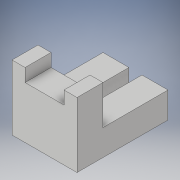
# Autodesk Inventor part: AddSub (1)
Saved by Autodesk Inventor 2019 (Build 230136000, 136)
## iProperties
Created: 2019-09-05
Part Number: AddSub (1)
Material: Generic
Document SubType Name: Modeling
Designer: IED8
Density: 1 g/cm^3
Appearance: Default
Author: IED8
Autodesk Inventor part; units mm, degrees
ref_plane "YZ Plane" through (0, 0, 0) normal (1, 0, 0) x (0, 1, 0)
ref_plane "XZ Plane" through (0, 0, 0) normal (0, 1, 0) x (-1, 0, 0)
ref_plane "XY Plane" through (0, 0, 0) normal (0, 0, 1) x (1, 0, 0)
sketch "Sketch1" plane through (0, 0, 0) normal (1, 0, 0) x (0, 1, 0)
  line L0 (0, 58.45) -> (0, -119.35)
  line L1 (0, -119.35) -> (50.8, -119.35)
  line L2 (50.8, -119.35) -> (50.8, 58.45)
  line L3 (50.8, 58.45) -> (0, 58.45)
  point P0 (0, 0)
  dimension "d0" = 177.8
  dimension "d1" = 50.8
  dimension "d2" = 177.8
  constraints: 8 end point, 2 vertical, 1 perpendicular
  measures "d0" distance of L0.start L0.end
  measures "d1" distance of L0.end L1.end
  measures "d2" distance of L1.end L2.end
extrude "Extrusion1" add sketch "Sketch1" along normal blind 127
sketch "Sketch2" plane through (0, 50.8, 58.45) normal (0, 1, 0) x (1, 0, 0)
  line L0 (0, 0) -> (0, 50.8)
  line L1 (0, 0) -> (0, 177.8) projected
  line L2 (0, 50.8) -> (127, 50.8)
  line L3 (127, 0) -> (127, 177.8) projected
  line L4 (127, 50.8) -> (127, 0)
  line L5 (0, 0) -> (127, 0) projected
  line L6 (127, 0) -> (0, 0)
  point P0 (0, 58.45)
  dimension "d5" = 50.8
  constraints: 8 end point, 2 point on line, 1 collinear, 1 perpendicular, 1 vertical
  measures "d5" distance of L0.start L0.end
extrude "Extrusion2" add sketch "Sketch2" along normal blind 76.2
sketch "Sketch3" plane through (0, 50.8, -119.35) normal (0, 1, 0) x (1, 0, 0)
  line L0 (0, 0) -> (127, 0) projected
  line L1 (50.7885, 0) -> (50.7885, -76.1988)
  line L2 (50.7885, -76.1988) -> (76.1885, -76.1988)
  line L3 (76.1885, -76.1988) -> (76.1885, 0)
  line L4 (50.7885, 0) -> (76.1885, 0)
  point P0 (0, -119.35)
  dimension "d8" = 25.4
  constraints: 8 end point, 3 perpendicular, 2 point on line, 1 vertical
  measures "d8" distance of L1.end L2.end
extrude "Extrusion3" cut sketch "Sketch3" against normal blind 50.8
sketch "Sketch4" plane through (127, 50.8, 7.65) normal (0, 0, -1) x (-1, 0, 0)
  line L0 (0, 76.2) -> (127, 76.2) projected
  line L1 (25.3885, 76.2) -> (25.3745, 50.7949)
  line L2 (25.3745, 50.7949) -> (101.5745, 50.7531)
  line L3 (101.5745, 50.7531) -> (101.5885, 76.2)
  line L4 (25.3885, 76.2) -> (101.5885, 76.2)
  point P0 (127, -50.8)
  dimension "d11" = 76.2
  constraints: 8 end point, 2 perpendicular, 2 point on line, 1 collinear
  measures "d11" distance of L1.end L2.end
extrude "Extrusion4" cut sketch "Sketch4" against normal blind 50.8
body "Solid1"
